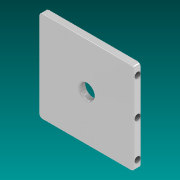
# Autodesk Inventor part: bevestegingsplaat axis5_6
Saved by Autodesk Inventor 2020 (Build 240168000, 168)
## iProperties
Created: 2020-05-25
Part Number: bevestegingsplaat axis5_6
Material: Generic
Document SubType Name: Modeling
Designer: stefa
Density: 1 g/cm^3
Appearance: Aluminum - Polished
Author: stefa
Autodesk Inventor part; units mm, degrees
ref_plane "YZ Plane" through (0, 0, 0) normal (1, 0, 0) x (0, 1, 0)
ref_plane "XZ Plane" through (0, 0, 0) normal (0, 1, 0) x (-1, 0, 0)
ref_plane "XY Plane" through (0, 0, 0) normal (0, 0, 1) x (1, 0, 0)
sketch "Sketch1" plane through (0, 0, 0) normal (0, 0, 1) x (1, 0, 0)
  line L0 (-26, -25) -> (26, -25)
  line L1 (26, -25) -> (26, 25)
  line L2 (26, 25) -> (-26, 25)
  line L3 (-26, 25) -> (-26, -25)
  line L4 (-26, -25) -> (26, 25) construction
  line L5 (26, -25) -> (-26, 25) construction
  circle A0 centre (0, 0) radius 4
  dimension "d0" = 52
  dimension "d1" = 50
  dimension "d2" = 8
  constraints: 12 end point, 2 midpoint, 2 parallel, 1 centre point, 1 coincident, 1 horizontal, 1 perpendicular
  measures "d0" distance of L2.end L1.end
  measures "d1" distance of L1.end L0.end
  measures "d2" diameter of A0
extrude "Extrusion1" add sketch "Sketch1" along normal mid plane 4
sketch "Sketch5" plane through (26, -25, 2) normal (1, 0, 0) x (0, 0, -1)
  point P0 (2, 25)
  point P1 (2, 25)
  point P2 (2, 45)
  point P3 (2, 5)
  dimension "d7" = 20
  dimension "d8" = 20
  constraints: 2 vertical alignment, 1 coincident
  measures "d7" distance of point (2, 5) point (2, 25)
  measures "d8" distance of point (2, 45) point (2, 25)
hole "Hole1" at (26, 0, 0) at (26, -20, 0) at (26, 20, 0) at (26, 0, 0) direction (-1, 0, 0) diameter 3.242 depth 11.8 tip angle 118 thread size "M4x0.7" class "6H" standard "ANSI Metric M Profile"
mirror "Mirror1" about plane through (0, 0, 0) normal (1, 0, 0) of "Hole1"
fillet "Fillet2" radius 0.5 8 edges at (0, -25, 2) (0, -25, -2) (0, 25, 2) (0, 25, -2) (26, 0, 2) (-26, 0, 2) (26, 0, -2) (-26, 0, -2)
fillet "Fillet3" radius 2 12 edges at (-25.8536, -24.8536, 1.8536) (-25.8536, -24.8536, -1.8536) (-26, -25, 0) (25.8536, -24.8536, 1.8536) (25.8536, -24.8536, -1.8536) (26, -25, 0) (25.8536, 24.8536, -1.8536) (25.8536, 24.8536, 1.8536) (26, 25, 0) (-25.8536, 24.8536, 1.8536) (-25.8536, 24.8536, -1.8536) (-26, 25, 0)
fillet "Fillet4" radius 1 2 edges at (-4, 0, 2) (-4, 0, -2)
equation "\"d8\" = d7"
body "Solid1"
